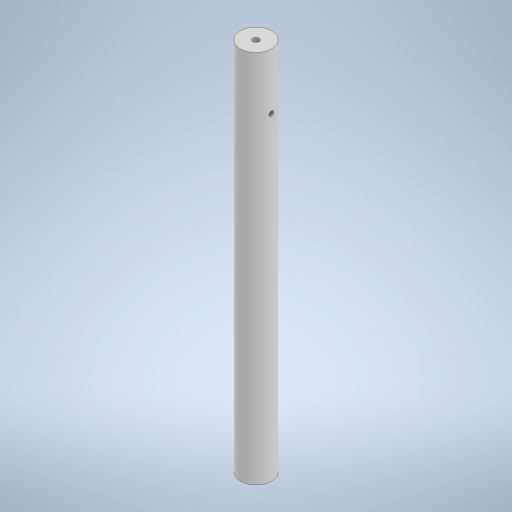
# Autodesk Inventor part: Вал
Saved by Autodesk Inventor 2023 (Build 270158000, 158)
## iProperties
Created: 2022-05-01
Part Number: Вал
Material: Типовые
Document SubType Name: Modeling
Designer: User
Density: 1 g/cm^3
Appearance: По умолчанию
Author: User
Autodesk Inventor part; units mm, degrees
ref_plane "YZ Plane" through (0, 0, 0) normal (1, 0, 0) x (0, 1, 0)
ref_plane "XZ Plane" through (0, 0, 0) normal (0, 1, 0) x (-1, 0, 0)
ref_plane "XY Plane" through (0, 0, 0) normal (0, 0, 1) x (1, 0, 0)
sketch "Эскиз1" plane through (0, 0, 0) normal (0, 1, 0) x (-1, 0, 0)
  circle A0 centre (0, 0) radius 12.5
  dimension "d0" = 25
  constraints: 1 centre point, 1 coincident
  measures "d0" diameter of A0
extrude "Выдавливание1" add sketch "Эскиз1" along normal blind 300
sketch "Эскиз2" plane through (0, 0, 0) normal (0, -1, 0) x (1, 0, 0)
  circle A0 centre (0, 0) radius 22.5
  line L0 (0, 0) -> (0, 4.5)
  line L1 (0, 0) -> (0, -4.5)
  dimension "d3" = 45
  dimension "d4" = 4.5
  dimension "d5" = 4.5
  constraints: 4 end point, 2 vertical, 1 centre point, 1 coincident
  measures "d3" diameter of A0
  measures "d4" distance of L0.start L0.end
  measures "d5" distance of L0.start L1.end
hole "Отверстие1" at (0, 0, 4.5) at (0, 0, -4.5) direction (0, 1, 0) diameter 2.459 depth 8 tip angle 118 thread size "M3x0.5" class "6H" standard "ISO Metric profile"
chamfer "Фаска1" distance 0.5 angle 45 2 edges at (0, 0, 5.7295) (0, 0, -3.2705)
sketch "Эскиз3" plane through (0, 300, 0) normal (0, 1, 0) x (1, 0, 0)
  circle A0 centre (0, 0) radius 2
  dimension "d16" = 4
  constraints: 1 centre point, 1 coincident
  measures "d16" diameter of A0
extrude "Выдавливание2" cut sketch "Эскиз3" against normal blind 10
sketch "Эскиз4" plane through (0, 0, 0) normal (1, 0, 0) x (0, 1, 0)
  line L0 (300, -12.5) -> (300, 12.5) projected
  line L1 (300, 0) -> (290, 0)
  circle A0 centre (290, 0) radius 1.5
  line L2 (300, 0) -> (250, 0)
  line L3 (250, 0) -> (255, 0)
  line L4 (255, 0) -> (245, 0)
  circle A1 centre (255, 0) radius 1.5
  circle A2 centre (245, 0) radius 1.5
  point P0 (0, 0)
  dimension "d29" = 10
  dimension "d30" = 3
  dimension "d35" = 50
  dimension "d36" = 5
  dimension "d37" = 10
  dimension "d38" = 3
  constraints: 8 end point, 3 centre point, 3 coincident, 2 horizontal, 2 point on line, 1 midpoint
  measures "d29" distance of L1.start L1.end
  measures "d30" diameter of A0
  measures "d35" distance of L1.start L2.end
  measures "d36" distance of L2.end L3.end
  measures "d37" distance of L3.end L4.end
  measures "d38" diameter of A1
extrude "Выдавливание3" cut sketch "Эскиз4" along normal mid plane 30.75 contours A1 L2 | L2 A1
chamfer "Фаска3" distance 0.5 angle 45 3 edges at (12.5, 253.5001, -0.0192) (-12.4097, 255.0001, 1.5) (-12.4097, 255.0013, -1.5)
chamfer "Фаска4" distance 0.5 angle 45 1 edges at (-2, 300, 0)
thread "Резьба3" size "M3x0.5" class "6H" standard "ANSI Metric M Profile" full length
